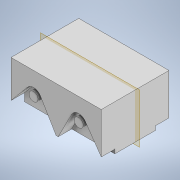
# Autodesk Inventor part: dog_body
Saved by Autodesk Inventor 2020 (Build 240168000, 168)
## iProperties
Created: 2020-12-19
Part Number: dog_body
Material: Generic
Document SubType Name: Modeling
Designer: frost
Density: 1 g/cm^3
Appearance: Default
Author: frost
Autodesk Inventor part; units mm, degrees
ref_plane "YZ Plane" through (0, 0, 0) normal (1, 0, 0) x (0, 1, 0)
ref_plane "XZ Plane" through (0, 0, 0) normal (0, 1, 0) x (-1, 0, 0)
ref_plane "XY Plane" through (0, 0, 0) normal (0, 0, 1) x (1, 0, 0)
sketch "Sketch1" plane through (0, 0, 0) normal (0, 0, 1) x (1, 0, 0)
  line L0 (20, -10) -> (-20, -10)
  line L1 (-20, -10) -> (-20, 10)
  line L2 (-20, 10) -> (20, 10)
  line L3 (20, 10) -> (20, -10)
  line L4 (20, -10) -> (-20, 10) construction
  line L5 (-20, -10) -> (20, 10) construction
  point P0 (0, 0)
  dimension "d0" = 40
  dimension "d1" = 20
  constraints: 12 end point, 2 midpoint, 2 parallel, 1 horizontal, 1 perpendicular
  measures "d0" distance of L1.end L2.end
  measures "d1" distance of L0.end L1.end
extrude "Extrusion1" add sketch "Sketch1" along normal mid plane 30
sketch "Sketch2" plane through (0, 0, 15) normal (0, 0, 1) x (1, 0, 0)
  arc A0 (-6.9896, 1.7854) -> (-12.6868, 2.243) centre (-10, 0) ccw
  line L0 (0, 0) -> (0, 12.7092)
  line L1 (-20, 10) -> (-20, -10) projected
  line L2 (-20, -6.5169) -> (-12.6868, 2.243)
  line L3 (-20, -10) -> (20, -10) projected
  line L4 (0, -10) -> (-6.9896, 1.7854)
  arc A1 (12.8699, 2.0034) -> (6.8274, 1.4781) centre (10, 0) ccw
  line L5 (0.8937, -10) -> (6.8274, 1.4781)
  line L6 (20, -10) -> (20, 10) projected
  line L7 (20, -8.2108) -> (12.8699, 2.0034)
  circle A2 centre (-10, 0) radius 2
  circle A3 centre (10, 0) radius 2
  line L8 (-5.9308, 0) -> (-6.5, 0)
  line L9 (-20, -6.5169) -> (-20, -10)
  line L10 (0, -10) -> (-20, -10)
  line L11 (0.8937, -10) -> (20, -10)
  line L12 (20, -8.2108) -> (20, -10)
  dimension "d4" = 7
  dimension "d5" = 10
  dimension "d6" = 4
  dimension "d7" = 4
  constraints: 20 end point, 4 centre point, 4 point on circle, 3 point on line, 3 tangent, 3 vertical, 2 coincident, 2 collinear, 1 horizontal, 1 midpoint, 1 symmetric about line, 1 other
  measures "d4" diameter of A0
  measures "d5" distance from line of L0 A0.centre
  measures "d6" diameter of A2
  measures "d7" diameter of A3
extrude "Extrusion2" cut sketch "Sketch2" against normal blind 6
ref_plane "Work Plane1" through (0, 0, 0) normal (0, 0, 1) x (1, 0, 0)
mirror "Mirror1" about plane through (0, 0, 0) normal (0, 0, 1) of "Extrusion2"
body "Solid1"
